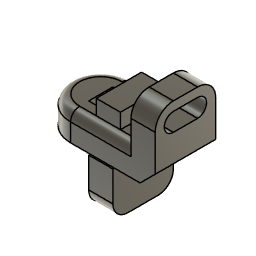
3Dprint 1 (Autodesk Fusion 360 design; units mm, degrees)
Autodesk Fusion 360 part; units mm, degrees
sketch "Sketch1" plane through (0, 0, 0) normal (0, 0, 1) x (1, 0, 0)
  line L0 (-28, 20) -> (0, 20)
  line L1 (0, 20) -> (0, 0)
  line L2 (0, 0) -> (-28, 0)
  arc A0 (-28, 20) -> (-28, 0) centre (-28, 10) ccw
  line L3 (-28, 14) -> (-8, 14)
  line L4 (-8, 6) -> (-28, 6)
  line L5 (-28, 14) -> (-28, 6)
  line L6 (-8, 20) -> (-8, 0)
  dimension "d1" = 28
  dimension "d3" = 28
  dimension "d4" = 10
  dimension "d6" = 20
  dimension "d15" = 20
  dimension "d17" = 8
  constraint horizontal L0
  constraint perpendicular L0 L1
  constraint perpendicular L1 L2
  constraint tangent L0 A0
  constraint perpendicular L4 L5
  constraint coincident L1.end L2.start
  constraint coincident L0 L6.start
  constraint coincident L2 L6.end
  constraint perpendicular L2 L6
  measures "d1" distance of L0.start L0.end
  measures "d3" distance of L1.end L2.end
  measures "d4" radius of A0
  measures "d6" distance of L3.start L3.end
  measures "d15" distance of L0.end L1.end
  measures "d17" distance of L3.start L4.end
extrude "Extrude1" add sketch "Sketch1" along normal blind 23 contours L0 L1 L2 L6 makes body 1
extrude "Extrude2" add sketch "Sketch1" along normal blind 9 contours L0 L2 A0 L3 L4 L5 L6 bodies 1
chamfer "Chamfer1" distance 5 angle 45 1 edges at (0, 10, 0) on bodies 1
fillet "Fillet1" radius 6 2 edges at (-4, 0, 23) (-4, 20, 23) on bodies 1
sketch "Sketch2" plane through (-8, 0, 0) normal (-1, 0, 0) x (0, -1, 0)
  arc A0 (-14, 23) -> (-20, 17) centre (-14, 17) ccw
  line L0 (-20, 17) -> (-20, 9)
  line L1 (-20, 9) -> (-14, 9)
  line L2 (-14, 9) -> (-14, 0)
  line L3 (-14, 0) -> (-6, 0)
  line L4 (-6, 0) -> (-6, 9)
  line L5 (-6, 9) -> (0, 9)
  line L6 (0, 9) -> (0, 17)
  arc A1 (0, 17) -> (-6, 23) centre (-6, 17) ccw
  line L7 (-6, 23) -> (-14, 23)
  line L8 (-14, 20) -> (-6, 20)
  line L9 (-6, 14) -> (-14, 14)
  arc A2 (-6.0011, 14) -> (-6, 20) centre (-6, 17) ccw
  arc A3 (-14, 20) -> (-14, 14) centre (-14, 17) ccw
  point P0 (-20, 0)
  dimension "d30" = 6
  dimension "d31" = 8
  constraint concentric A1 A2
  constraint tangent L8 A2
  constraint coincident L9.start A2
  constraint coincident L9.end A3
  constraint tangent L9 A3
  constraint coincident L9 A2.start
  constraint coincident L9 A3.end
  measures "d30" distance of L8 L9
  measures "d31" distance of A1.centre A0.centre
extrude "Extrude3" cut sketch "Sketch2" against normal through all contours L8 L9 A2 A3 bodies 1
fillet "Fillet2" radius 3 3 edges at (-18, 20, 9) (-38, 10, 9) (-18, 0, 9) on bodies 1
sketch "Sketch3" plane through (0, 0, 0) normal (0, 1, 0) x (1, 0, 0)
  line L0 (0, 0) -> (20, 0)
  line L1 (20, 0) -> (20, 15)
  line L2 (20, 15) -> (13.5, 15)
  line L3 (13.5, 15) -> (13.5, 25)
  line L4 (13.5, 25) -> (17.5, 25)
  line L5 (17.5, 25) -> (17.5, 30)
  line L6 (17.5, 30) -> (2.5, 30)
  line L7 (2.5, 30) -> (2.5, 25)
  line L8 (2.5, 25) -> (6.5, 25)
  line L9 (6.5, 25) -> (6.5, 15)
  line L10 (6.5, 15) -> (0, 15)
  line L11 (0, 15) -> (0, 0)
  dimension "d40" = 20
  dimension "d41" = 15
  dimension "d43" = 10
  dimension "d45" = 5
  dimension "d46" = 15
  dimension "d56" = 6.5
  dimension "d57" = 6.5
  dimension "d58" = 4
  dimension "d59" = 4
  constraint coincident L0.start L11.end
  constraint perpendicular L1 L2
  constraint perpendicular L3 L4
  constraint perpendicular L4 L5
  constraint perpendicular L3 L6
  constraint perpendicular L6 L7
  constraint perpendicular L7 L8
  constraint perpendicular L6 L9
  constraint perpendicular L9 L10
  constraint perpendicular L0 L11
  constraint horizontal L0
  constraint vertical L1
  constraint horizontal L10
  constraint collinear L4 L8
  constraint collinear L2 L10
  measures "d40" distance of L0.start L0.end
  measures "d41" distance of L0.end L1.end
  measures "d43" distance of L2.end L3.end
  measures "d45" distance of L4.end L5.end
  measures "d46" distance of L5.end L6.end
  measures "d56" distance of L1.end L2.end
  measures "d57" distance of L9.end L10.end
  measures "d58" distance of L7.end L8.end
  measures "d59" distance of L3.end L4.end
extrude "Extrude4" add sketch "Sketch3" along normal blind 8 separate body makes body 2
move_body "Move1" bodies 2 to x (1, 0, 0) y (0, 1, 0) z (0, 0, 1) at (10, 0, 30)
fillet "Fillet3" radius 5 2 edges at (30, 4, 30) (10, 4, 30) on bodies 2
sketch "Sketch5" plane through (0, 0, 0) normal (0, -1, 0) x (1, 0, 0)
  arc A0 (15, 30) -> (10, 25) centre (15, 25) ccw
  line L0 (10, 25) -> (10, 15)
  line L1 (10, 15) -> (16.5, 15)
  line L2 (16.5, 15) -> (16.5, 5)
  line L3 (16.5, 5) -> (12.5, 5)
  line L4 (12.5, 5) -> (12.5, 0)
  line L5 (12.5, 0) -> (27.5, 0)
  line L6 (27.5, 0) -> (27.5, 5)
  line L7 (27.5, 5) -> (23.5, 5)
  line L8 (23.5, 5) -> (23.5, 15)
  line L9 (23.5, 15) -> (30, 15)
  line L10 (30, 15) -> (30, 25)
  arc A1 (30, 25) -> (25, 30) centre (25, 25) ccw
  line L11 (25, 30) -> (15, 30)
  line L12 (13.0742, 16.0006) -> (27.1762, 15.8861) construction
  line L13 (27.1762, 15.8861) -> (27.2684, 27.2361) construction
  line L14 (27.2684, 27.2361) -> (13.1664, 27.3507) construction
  line L15 (13.1664, 27.3507) -> (13.0742, 16.0006) construction
  dimension "d53" = 10
  text T0 "01" font "Arial" height 10 align left top in box 14.1025 x 11.3504 at (13.0742, 16.0006) x (0.999967, -0.008124) y (0.008124, 0.999967) spacing 1
sketch "Sketch6" plane through (0, 0, 0) normal (0, -1, 0) x (1, 0, 0)
extrude "Extrude5" cut sketch "Sketch5" against normal blind 1 text T0 bodies 2
move_body "Move2" bodies 2 to x (0, 1, 0) y (1, 0, 0) z (0, 0, -1) at (10, -35, 25)
copy_body "Body->Comp1" bodies 1 removing the originals makes body 3 in component "Component"
copy_body "Body->Comp2" bodies 2 removing the originals makes body 4 in component "Component'"
component "Component" placed x (1, 0, 0) y (0, 1, 0) z (0, 0, 1) at (0, 0, 0)
component "Component'" placed x (1, 0, 0) y (0, 1, 0) z (0, 0, 1) at (-32, 25, -10.5)
